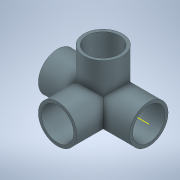
# Autodesk Inventor part: hoek vierweg
Saved by Autodesk Inventor 2020.2 (Build 242310000, 310)
## iProperties
Created: 2019-11-27
Part Number: hoek vierweg
Material: ABS Plastic
Document SubType Name: Modeling
Designer: Gebruiker
Density: 1.06 g/cm^3
Appearance: Lead
Author: Gebruiker
Autodesk Inventor part; units mm, degrees
sketch "Sketch1" plane through (0, 0, 0) normal (0, 1, 0) x (-1, 0, 0)
  line L0 (0, 0) -> (0, 30)
  line L1 (0, 0) -> (-30, 0)
  dimension "d0" = 30
  dimension "d1" = 30
  constraints: 4 end point, 1 horizontal, 1 vertical
  measures "d0" distance of L0.start L0.end
  measures "d1" distance of L0.start L1.end
ref_plane "Work Plane1" through (0, 0, 30) normal (0, 0, 1) x (1, 0, 0)
sketch "Sketch2" plane through (0, 0, 30) normal (0, 0, 1) x (1, 0, 0)
  circle A0 centre (0, 0) radius 12.65
  dimension "d2" = 25.3
  constraints: 1 centre point, 1 coincident
  measures "d2" diameter of A0
sketch "Sketch3" plane through (0, 0, 0) normal (0, 1, 0) x (-1, 0, 0)
  line L0 (0, 0) -> (0, 30) projected
sweep "Sweep1" add profiles "Sketch2" path "Sketch3"
sketch "Sketch4" plane through (0, 0, 0) normal (1, 0, 0) x (0, 1, 0)
  line L0 (0, 0) -> (30, 0)
  dimension "d5" = 30
  constraints: 2 end point, 1 horizontal
  measures "d5" distance of L0.start L0.end
ref_plane "Work Plane2" through (0, 30, 0) normal (0, 1, 0) x (-1, 0, 0)
sketch "Sketch5" plane through (0, 30, 0) normal (0, 1, 0) x (-1, 0, 0)
  circle A0 centre (0, 0) radius 12.65
  dimension "d6" = 25.3
  constraints: 1 centre point, 1 coincident
  measures "d6" diameter of A0
sweep "Sweep2" add profiles "Sketch5" path "Sketch4" separate body
sketch "Sketch6" plane through (0, 0, 0) normal (0, 1, 0) x (-1, 0, 0)
  line L0 (0, 0) -> (-30, 0) projected
ref_plane "Work Plane3" through (30, 0, 0) normal (1, 0, 0) x (0, 1, 0)
sketch "Sketch12" plane through (0, 0, 0) normal (1, 0, 0) x (0, 1, 0)
  circle A0 centre (0, 0) radius 12.65
  dimension "d15" = 25.3
  constraints: 1 centre point, 1 coincident
  measures "d15" diameter of A0
extrude "Extrusion1" add sketch "Sketch12" along normal mid plane 60 bodies 1
sketch "Sketch14" plane through (0, 30, 0) normal (0, 1, 0) x (1, 0, 0)
  line L0 (-12.65, -12.65) -> (0, 0) projected
  circle A0 centre (0, 0) radius 10.65
  dimension "d21" = 21.3
  constraints: 1 centre point, 1 coincident
  measures "d21" diameter of A0
sketch "Sketch18" plane through (-30, 0, 0) normal (-1, 0, 0) x (0, 0, 1)
  circle A0 centre (0, 0) radius 10.65
  dimension "d30" = 21.3
  constraints: 1 centre point, 1 coincident
  measures "d30" diameter of A0
extrude "Extrusion7" cut sketch "Sketch18" against normal blind 15 bodies 1
sketch "Sketch19" plane through (30, 0, 0) normal (1, 0, 0) x (0, 0, -1)
  circle A0 centre (0, 0) radius 10.65
  dimension "d33" = 21.3
  constraints: 1 centre point, 1 coincident
  measures "d33" diameter of A0
extrude "Extrusion8" cut sketch "Sketch19" against normal blind 15 bodies 1
sketch "Sketch20" plane through (0, 0, 30) normal (0, 0, 1) x (1, 0, 0)
  circle A0 centre (0, 0) radius 10.65
  dimension "d36" = 21.3
  constraints: 1 centre point, 1 coincident
  measures "d36" diameter of A0
extrude "Extrusion9" cut sketch "Sketch20" against normal blind 15 bodies 1
extrude "Extrusion10" cut sketch "Sketch14" against normal blind 15 bodies 2
equation "\"d1\" = d0"
body "Solid1"
body "Solid2"
